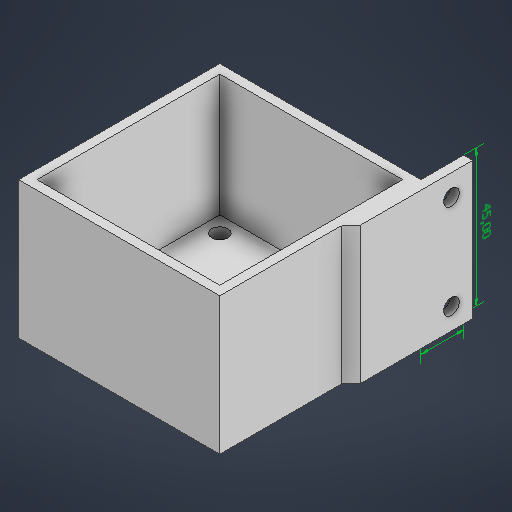
# Autodesk Inventor part: soporte motor
Saved by Autodesk Inventor 2026.1 (Build 301233020, 233B)
## iProperties
Created: 2025-11-23
Part Number: soporte motor
Material: Generic
Document SubType Name: Modeling
Designer: Tito Luyo Murata
Density: 1 g/cm^3
Appearance: Default
Author: Tito Luyo Murata
Autodesk Inventor part; units mm, degrees
ref_plane "YZ Plane" through (0, 0, 0) normal (1, 0, 0) x (0, 1, 0)
ref_plane "XZ Plane" through (0, 0, 0) normal (0, 1, 0) x (-1, 0, 0)
ref_plane "XY Plane" through (0, 0, 0) normal (0, 0, 1) x (1, 0, 0)
sketch "Sketch1" plane through (0, 0, 0) normal (0, 1, 0) x (-1, 0, 0)
  line L0 (0, 0) -> (60, 0)
  line L1 (60, 0) -> (60, -60)
  line L2 (60, -60) -> (0, -60)
  line L3 (0, -60) -> (0, 0)
  line L4 (-3, -63) -> (63, -63)
  line L5 (63, -63) -> (63, 3)
  line L6 (63, 3) -> (-3, 3)
  line L7 (-3, 3) -> (-3, -63)
  dimension "d0" = 60
  dimension "d1" = 60
  dimension "d2" = 3
  constraints: 16 end point, 4 parallel, 2 perpendicular, 1 horizontal, 3 other
  measures "d0" distance of L1.end L2.end
  measures "d1" distance of L0.end L1.end
  measures "d2" distance between parallel lines of L2 L4
extrude "Extrusion1" add sketch "Sketch1" along normal blind 40
sketch "Sketch2" plane through (0, 0, 0) normal (0, -1, 0) x (1, 0, 0)
  line L0 (-63, -63) -> (-63, 3) projected
  line L1 (-63, 3) -> (3, 3)
  line L2 (3, 3) -> (3, -63)
  line L3 (3, -63) -> (-63, -63)
  line L4 (-63, -63) -> (-63, 3)
  point P0 (0, 0)
  dimension "d5" = 66
  dimension "d6" = 66
  constraints: 8 end point, 2 parallel, 1 horizontal, 1 perpendicular
  measures "d5" distance of L2.end L3.end
  measures "d6" distance of L1.end L2.end
extrude "Extrusion2" add sketch "Sketch2" along normal blind 5
sketch "Sketch3" plane through (0, -5, 0) normal (0, -1, 0) x (1, 0, 0)
  line L0 (20, -30) -> (-80, -30) construction
  line L1 (-30, 20) -> (-30, -80) construction
  circle A0 centre (-54.75, -5.25) radius 2.65
  circle A1 centre (-5.25, -5.25) radius 2.65
  circle A2 centre (-54.75, -54.75) radius 2.65
  circle A3 centre (-5.25, -54.75) radius 2.65
  point P0 (0, 0)
  dimension "d9" = 100
  dimension "d10" = 30
  dimension "d11" = 100
  dimension "d12" = 30
  dimension "d13" = 24.75
  dimension "d14" = 24.75
  dimension "d15" = 5.3
  dimension "d18" = 49.5
  dimension "d21" = 49.5
  constraints: 4 centre point, 4 end point, 2 horizontal, 2 vertical, 6 other
  measures "d9" distance of L0.start L0.end
  measures "d10" distance from line of point (0, 0) L0
  measures "d11" distance of L1.start L1.end
  measures "d12" distance from line of point (0, 0) L1
  measures "d13" distance from line of L1 A0.centre
  measures "d14" distance from line of L0 A0.centre
  measures "d15" diameter of A0
  measures "d18" distance of A0.centre A1.centre
  measures "d21" distance of A0.centre A2.centre
extrude "Extrusion3" cut sketch "Sketch3" against normal blind 5
sketch "Sketch4" plane through (0, 0, 0) normal (0, 1, 0) x (1, 0, 0)
  line L0 (20, 30) -> (-80, 30) construction
  line L1 (0, 0) -> (-60, 0) construction
  line L2 (-30, -20) -> (-30, 80) construction
  line L3 (0, 60) -> (0, 0) construction
  circle A0 centre (-30, 20) radius 12.5
  dimension "d26" = 100
  dimension "d27" = 30
  dimension "d28" = 100
  dimension "d29" = 30
  dimension "d30" = 25
  dimension "d31" = 10
  constraints: 4 end point, 1 centre point, 1 horizontal, 1 point on line, 1 vertical
  measures "d26" distance of L0.start L0.end
  measures "d27" distance between parallel lines of L1 L0
  measures "d28" distance of L2.start L2.end
  measures "d29" distance between parallel lines of L3 L2
  measures "d30" diameter of A0
  measures "d31" distance from line of L0 A0.centre
extrude "Extrusion4" cut sketch "Sketch4" against normal blind 3.3
sketch "Sketch5" plane through (-30, -3.3, -20) normal (0, 1, 0) x (1, 0, 0)
  circle A0 centre (0, 0) radius 4.25
  point P0 (30, -20)
  dimension "d34" = 8.5
  constraints: 1 centre point
  measures "d34" diameter of A0
extrude "Extrusion5" cut sketch "Sketch5" against normal blind 2
sketch "Sketch6" plane through (3, 40, 3) normal (1, 0, 0) x (0, 0, -1)
  line L0 (66, 0) -> (0, 0) projected
  line L1 (40, 0) -> (80, 0)
  line L2 (80, 0) -> (80, -45)
  line L3 (80, -45) -> (40, -45)
  line L4 (40, -45) -> (40, 0)
  point P0 (3, -40)
  dimension "d37" = 40
  dimension "d38" = 40
  constraints: 8 end point, 2 parallel, 1 horizontal, 1 perpendicular, 1 point on line
  measures "d37" distance of L2.end L3.end
  measures "d38" distance from line of L0.end L4
extrude "Extrusion6" add sketch "Sketch6" along normal blind 3
chamfer "Chamfer1" distance 3 angle 45 1 edges at (6, 17.5, -37)
sketch "Sketch7" plane through (3, 40, 3) normal (-1, 0, 0) x (0, 0, 1)
  circle A0 centre (-73, -38) radius 2.6
  line L0 (-80, -45) -> (-80, 0) projected
  line L1 (-66, -45) -> (-80, -45) projected
  circle A1 centre (-73, -7) radius 2.6
  line L2 (-80, 0) -> (-66, 0) projected
  point P0 (-3, -40)
  dimension "d44" = 5.2
  dimension "d51" = 7
  dimension "d52" = 7
  dimension "d53" = 5.2
  dimension "d54" = 7
  dimension "d55" = 7
  constraints: 2 centre point
  measures "d44" diameter of A0
  measures "d51" distance from line of L0 A0.centre
  measures "d52" distance from line of L1 A0.centre
  measures "d53" diameter of A1
  measures "d54" distance from line of L2 A1.centre
  measures "d55" distance from line of L0 A1.centre
extrude "Extrusion7" cut sketch "Sketch7" against normal blind 3
body "Solid1"
